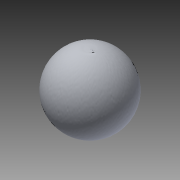
# Autodesk Inventor part: ping_pong_ball
Saved by Autodesk Inventor 2013 (Build 170138000, 138)
## iProperties
Created: 2013-07-24
Part Number: ping_pong_ball
Material: Generic
Document SubType Name: Modeling
Designer: dkboone
Density: 1 g/cm^3
Author: dkboone
Autodesk Inventor part; units mm, degrees
ref_plane "YZ Plane" through (0, 0, 0) normal (1, 0, 0) x (0, 1, 0)
ref_plane "XZ Plane" through (0, 0, 0) normal (0, 1, 0) x (-1, 0, 0)
ref_plane "XY Plane" through (0, 0, 0) normal (0, 0, 1) x (1, 0, 0)
sketch "Sketch1" plane through (0, 0, 0) normal (0, 1, 0) x (-1, 0, 0)
  circle A0 centre (0, 0) radius 20
  line L0 (16.3846, 11.4692) -> (-16.3846, -11.4692)
  dimension "d1" = 40
  constraints: 2 end point, 2 point on circle, 1 centre point, 1 coincident, 1 midpoint
  measures "d1" diameter of A0
revolve "Revolution1" add sketch "Sketch1" angle 360 about axis through (-16.3846, 0, 11.4692) along (0.8192319, 0, -0.5734624) picked at (-4.4535, 4.9609) contours L0 A0
body "Solid1"
